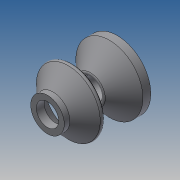
# Autodesk Inventor part: player
Saved by Autodesk Inventor 2015 SP1 (Build 190203100, 203)
## iProperties
Created: 2015-12-28
Part Number: player
Material: Generic
Document SubType Name: Modeling
Designer: Florian
Density: 1 g/cm^3
Appearance: Default
Author: Florian
Autodesk Inventor part; units mm, degrees
ref_plane "YZ Plane" through (0, 0, 0) normal (1, 0, 0) x (0, 1, 0)
ref_plane "XZ Plane" through (0, 0, 0) normal (0, 1, 0) x (-1, 0, 0)
ref_plane "XY Plane" through (0, 0, 0) normal (0, 0, 1) x (1, 0, 0)
sketch "Sketch1" plane through (0, 0, 0) normal (0, 0, 1) x (1, 0, 0)
  line L0 (10, 0) -> (15, 0)
  line L1 (15, 0) -> (15, 5)
  line L2 (15, 5) -> (30, 20)
  line L3 (30, 20) -> (26.4645, 23.5355)
  line L4 (26.4645, 23.5355) -> (10, 7.0711)
  line L5 (10, 7.0711) -> (10, 0)
  line L6 (30, 55.3553) -> (10.718, 36.0733)
  line L7 (10.718, 36.0733) -> (0, 76.0733)
  line L8 (0, 0) -> (0, 76.0733)
  line L9 (30, 55.3553) -> (30, 62.4264)
  line L10 (30, 62.4264) -> (19.3934, 51.8198)
  line L11 (19.3934, 51.8198) -> (0, 76.0733)
  dimension "d0" = 45
  dimension "d1" = 20
  dimension "d2" = 5
  dimension "d3" = 5
  dimension "d4" = 5
  dimension "d5" = 15
  dimension "d7" = 20
  dimension "d8" = 60
  dimension "d9" = 5
  dimension "d10" = 15
  dimension "d14" = 40
  constraints: 24 end point, 3 parallel, 2 perpendicular, 2 vertical, 1 horizontal, 1 point on line, 1 vertical alignment
  measures "d0" angle of L2 L8
  measures "d1" diameter of L5 L8
  measures "d2" distance between parallel lines of L5 L1
  measures "d3" distance of L0.end L1.end
  measures "d4" distance between parallel lines of L2 L4
  measures "d5" horizontal distance of L1.end L2.end
  measures "d7" distance between parallel lines of L6 L4
  measures "d8" angle of L6 L7
  measures "d9" distance between parallel lines of L6 L10
  measures "d10" distance of L9.end L10.end
  measures "d14" vertical distance of L7.end L6.end
revolve "Revolution1" add sketch "Sketch1" angle 360 about axis through (0, 0, 0) along (0, 1, 0)
fillet "Fillet1" radius 2 3 edges at (-30, 20, 0) (-26.4645, 23.5355, 0) (-10.718, 36.0733, 0)
fillet "Fillet2" radius 5 1 edges at (-19.3934, 51.8198, 0)
equation "\"d4\" = d2"
equation "\"d7\" = d1"
equation "\"d9\" = d2"
body "Solid1"
